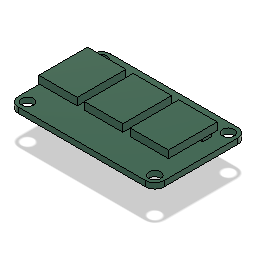
Button_PCB (Autodesk Fusion 360 design; units mm, degrees)
Autodesk Fusion 360 part; units mm, degrees
sketch "Sketch1" plane through (0, 0, 0) normal (0, 1, 0) x (1, 0, 0)
  line L0 (8.7286, -24.1072) -> (8.8714, -24.1548)
  line L1 (8.8714, -24.1548) -> (9.1095, -24.1548)
  line L2 (9.1095, -24.1548) -> (9.2048, -24.1072)
  line L3 (9.2048, -24.1072) -> (9.2524, -24.0595)
  line L4 (9.2524, -24.0595) -> (9.3, -23.9643)
  line L5 (9.3, -23.9643) -> (9.3, -23.8691)
  line L6 (9.3, -23.8691) -> (9.2524, -23.7738)
  line L7 (9.2524, -23.7738) -> (9.2048, -23.7262)
  line L8 (9.2048, -23.7262) -> (9.1095, -23.6786)
  line L9 (9.1095, -23.6786) -> (8.919, -23.631)
  line L10 (8.919, -23.631) -> (8.8238, -23.5833)
  line L11 (8.8238, -23.5833) -> (8.7762, -23.5357)
  line L12 (8.7762, -23.5357) -> (8.7286, -23.4405)
  line L13 (8.7286, -23.4405) -> (8.7286, -23.3453)
  line L14 (8.7286, -23.3453) -> (8.7762, -23.25)
  line L15 (8.7762, -23.25) -> (8.8238, -23.2024)
  line L16 (8.8238, -23.2024) -> (8.919, -23.1548)
  line L17 (8.919, -23.1548) -> (9.1571, -23.1548)
  line L18 (9.1571, -23.1548) -> (9.3, -23.2024)
  line L19 (10.1571, -23.4881) -> (10.1571, -24.1548)
  line L20 (9.7286, -23.4881) -> (9.7286, -24.0119)
  line L21 (9.7286, -24.0119) -> (9.7762, -24.1072)
  line L22 (9.7762, -24.1072) -> (9.8714, -24.1548)
  line L23 (9.8714, -24.1548) -> (10.0143, -24.1548)
  line L24 (10.0143, -24.1548) -> (10.1095, -24.1072)
  line L25 (10.1095, -24.1072) -> (10.1571, -24.0595)
  line L26 (10.6333, -23.4881) -> (10.6333, -24.1548)
  line L27 (10.6333, -23.5833) -> (10.681, -23.5357)
  line L28 (10.681, -23.5357) -> (10.7762, -23.4881)
  line L29 (10.7762, -23.4881) -> (10.919, -23.4881)
  line L30 (10.919, -23.4881) -> (11.0143, -23.5357)
  line L31 (11.0143, -23.5357) -> (11.0619, -23.631)
  line L32 (11.0619, -23.631) -> (11.0619, -24.1548)
  line L33 (11.5381, -24.1548) -> (11.5381, -23.4881)
  line L34 (11.5381, -23.6786) -> (11.5857, -23.5833)
  line L35 (11.5857, -23.5833) -> (11.6333, -23.5357)
  line L36 (11.6333, -23.5357) -> (11.7286, -23.4881)
  line L37 (11.7286, -23.4881) -> (11.8238, -23.4881)
  line L38 (12.1571, -24.1548) -> (12.1571, -23.4881)
  line L39 (12.1571, -23.1548) -> (12.1095, -23.2024)
  line L40 (12.1095, -23.2024) -> (12.1571, -23.25)
  line L41 (12.1571, -23.25) -> (12.2048, -23.2024)
  line L42 (12.2048, -23.2024) -> (12.1571, -23.1548)
  line L43 (12.1571, -23.1548) -> (12.1571, -23.25)
  line L44 (12.5857, -24.1072) -> (12.681, -24.1548)
  line L45 (12.681, -24.1548) -> (12.8714, -24.1548)
  line L46 (12.8714, -24.1548) -> (12.9667, -24.1072)
  line L47 (12.9667, -24.1072) -> (13.0143, -24.0119)
  line L48 (13.0143, -24.0119) -> (13.0143, -23.9643)
  line L49 (13.0143, -23.9643) -> (12.9667, -23.8691)
  line L50 (12.9667, -23.8691) -> (12.8714, -23.8214)
  line L51 (12.8714, -23.8214) -> (12.7286, -23.8214)
  line L52 (12.7286, -23.8214) -> (12.6333, -23.7738)
  line L53 (12.6333, -23.7738) -> (12.5857, -23.6786)
  line L54 (12.5857, -23.6786) -> (12.5857, -23.631)
  line L55 (12.5857, -23.631) -> (12.6333, -23.5357)
  line L56 (12.6333, -23.5357) -> (12.7286, -23.4881)
  line L57 (12.7286, -23.4881) -> (12.8714, -23.4881)
  line L58 (12.8714, -23.4881) -> (12.9667, -23.5357)
  line L59 (13.8238, -24.1072) -> (13.7286, -24.1548)
  line L60 (13.7286, -24.1548) -> (13.5381, -24.1548)
  line L61 (13.5381, -24.1548) -> (13.4429, -24.1072)
  line L62 (13.4429, -24.1072) -> (13.3952, -24.0119)
  line L63 (13.3952, -24.0119) -> (13.3952, -23.631)
  line L64 (13.3952, -23.631) -> (13.4429, -23.5357)
  line L65 (13.4429, -23.5357) -> (13.5381, -23.4881)
  line L66 (13.5381, -23.4881) -> (13.7286, -23.4881)
  line L67 (13.7286, -23.4881) -> (13.8238, -23.5357)
  line L68 (13.8238, -23.5357) -> (13.8714, -23.631)
  line L69 (13.8714, -23.631) -> (13.8714, -23.7262)
  line L70 (13.8714, -23.7262) -> (13.3952, -23.8214)
  line L71 (15.0143, -23.8691) -> (15.4905, -23.8691)
  line L72 (14.919, -24.1548) -> (15.2524, -23.1548)
  line L73 (15.2524, -23.1548) -> (15.5857, -24.1548)
  line L74 (16.0619, -24.1548) -> (15.9667, -24.1072)
  line L75 (15.9667, -24.1072) -> (15.919, -24.0119)
  line L76 (15.919, -24.0119) -> (15.919, -23.1548)
  line L77 (16.8714, -24.1548) -> (16.8714, -23.631)
  line L78 (16.8714, -23.631) -> (16.8238, -23.5357)
  line L79 (16.8238, -23.5357) -> (16.7286, -23.4881)
  line L80 (16.7286, -23.4881) -> (16.5381, -23.4881)
  line L81 (16.5381, -23.4881) -> (16.4429, -23.5357)
  line L82 (16.8714, -24.1072) -> (16.7762, -24.1548)
  line L83 (16.7762, -24.1548) -> (16.5381, -24.1548)
  line L84 (16.5381, -24.1548) -> (16.4429, -24.1072)
  line L85 (16.4429, -24.1072) -> (16.3952, -24.0119)
  line L86 (16.3952, -24.0119) -> (16.3952, -23.9167)
  line L87 (16.3952, -23.9167) -> (16.4429, -23.8214)
  line L88 (16.4429, -23.8214) -> (16.5381, -23.7738)
  line L89 (16.5381, -23.7738) -> (16.7762, -23.7738)
  line L90 (16.7762, -23.7738) -> (16.8714, -23.7262)
  line L91 (17.3476, -24.1548) -> (17.3476, -23.4881)
  line L92 (17.3476, -23.6786) -> (17.3952, -23.5833)
  line L93 (17.3952, -23.5833) -> (17.4429, -23.5357)
  line L94 (17.4429, -23.5357) -> (17.5381, -23.4881)
  line L95 (17.5381, -23.4881) -> (17.6333, -23.4881)
  line L96 (17.9667, -24.1548) -> (17.9667, -23.4881)
  line L97 (17.9667, -23.5833) -> (18.0143, -23.5357)
  line L98 (18.0143, -23.5357) -> (18.1095, -23.4881)
  line L99 (18.1095, -23.4881) -> (18.2524, -23.4881)
  line L100 (18.2524, -23.4881) -> (18.3476, -23.5357)
  line L101 (18.3476, -23.5357) -> (18.3952, -23.631)
  line L102 (18.3952, -23.631) -> (18.3952, -24.1548)
  line L103 (18.3952, -23.631) -> (18.4429, -23.5357)
  line L104 (18.4429, -23.5357) -> (18.5381, -23.4881)
  line L105 (18.5381, -23.4881) -> (18.681, -23.4881)
  line L106 (18.681, -23.4881) -> (18.7762, -23.5357)
  line L107 (18.7762, -23.5357) -> (18.8238, -23.631)
  line L108 (18.8238, -23.631) -> (18.8238, -24.1548)
  line L109 (19.919, -23.1548) -> (20.2524, -24.1548)
  line L110 (20.2524, -24.1548) -> (20.5857, -23.1548)
  line L111 (20.8238, -23.1548) -> (21.4429, -23.1548)
  line L112 (21.4429, -23.1548) -> (21.1095, -23.5357)
  line L113 (21.1095, -23.5357) -> (21.2524, -23.5357)
  line L114 (21.2524, -23.5357) -> (21.3476, -23.5833)
  line L115 (21.3476, -23.5833) -> (21.3952, -23.631)
  line L116 (21.3952, -23.631) -> (21.4429, -23.7262)
  line L117 (21.4429, -23.7262) -> (21.4429, -23.9643)
  line L118 (21.4429, -23.9643) -> (21.3952, -24.0595)
  line L119 (21.3952, -24.0595) -> (21.3476, -24.1072)
  line L120 (21.3476, -24.1072) -> (21.2524, -24.1548)
  line L121 (21.2524, -24.1548) -> (20.9667, -24.1548)
  line L122 (20.9667, -24.1548) -> (20.8714, -24.1072)
  line L123 (20.8714, -24.1072) -> (20.8238, -24.0595)
  line L124 (21.8714, -24.0595) -> (21.919, -24.1072)
  line L125 (21.919, -24.1072) -> (21.8714, -24.1548)
  line L126 (21.8714, -24.1548) -> (21.8238, -24.1072)
  line L127 (21.8238, -24.1072) -> (21.8714, -24.0595)
  line L128 (21.8714, -24.0595) -> (21.8714, -24.1548)
  line L129 (21.8714, -23.5357) -> (21.919, -23.5833)
  line L130 (21.919, -23.5833) -> (21.8714, -23.631)
  line L131 (21.8714, -23.631) -> (21.8238, -23.5833)
  line L132 (21.8238, -23.5833) -> (21.8714, -23.5357)
  line L133 (21.8714, -23.5357) -> (21.8714, -23.631)
  line L134 (23.4429, -23.631) -> (23.5857, -23.6786)
  line L135 (23.5857, -23.6786) -> (23.6333, -23.7262)
  line L136 (23.6333, -23.7262) -> (23.681, -23.8214)
  line L137 (23.681, -23.8214) -> (23.681, -23.9643)
  line L138 (23.681, -23.9643) -> (23.6333, -24.0595)
  line L139 (23.6333, -24.0595) -> (23.5857, -24.1072)
  line L140 (23.5857, -24.1072) -> (23.4905, -24.1548)
  line L141 (23.4905, -24.1548) -> (23.1095, -24.1548)
  line L142 (23.1095, -24.1548) -> (23.1095, -23.1548)
  line L143 (23.1095, -23.1548) -> (23.4429, -23.1548)
  line L144 (23.4429, -23.1548) -> (23.5381, -23.2024)
  line L145 (23.5381, -23.2024) -> (23.5857, -23.25)
  line L146 (23.5857, -23.25) -> (23.6333, -23.3453)
  line L147 (23.6333, -23.3453) -> (23.6333, -23.4405)
  line L148 (23.6333, -23.4405) -> (23.5857, -23.5357)
  line L149 (23.5857, -23.5357) -> (23.5381, -23.5833)
  line L150 (23.5381, -23.5833) -> (23.4429, -23.631)
  line L151 (23.4429, -23.631) -> (23.1095, -23.631)
  line L152 (24.5381, -23.4881) -> (24.5381, -24.1548)
  line L153 (24.1095, -23.4881) -> (24.1095, -24.0119)
  line L154 (24.1095, -24.0119) -> (24.1571, -24.1072)
  line L155 (24.1571, -24.1072) -> (24.2524, -24.1548)
  line L156 (24.2524, -24.1548) -> (24.3952, -24.1548)
  line L157 (24.3952, -24.1548) -> (24.4905, -24.1072)
  line L158 (24.4905, -24.1072) -> (24.5381, -24.0595)
  line L159 (24.8714, -23.4881) -> (25.2524, -23.4881)
  line L160 (25.0143, -23.1548) -> (25.0143, -24.0119)
  line L161 (25.0143, -24.0119) -> (25.0619, -24.1072)
  line L162 (25.0619, -24.1072) -> (25.1571, -24.1548)
  line L163 (25.1571, -24.1548) -> (25.2524, -24.1548)
  line L164 (25.4429, -23.4881) -> (25.8238, -23.4881)
  line L165 (25.5857, -23.1548) -> (25.5857, -24.0119)
  line L166 (25.5857, -24.0119) -> (25.6333, -24.1072)
  line L167 (25.6333, -24.1072) -> (25.7286, -24.1548)
  line L168 (25.7286, -24.1548) -> (25.8238, -24.1548)
  line L169 (26.3, -24.1548) -> (26.2048, -24.1072)
  line L170 (26.2048, -24.1072) -> (26.1571, -24.0595)
  line L171 (26.1571, -24.0595) -> (26.1095, -23.9643)
  line L172 (26.1095, -23.9643) -> (26.1095, -23.6786)
  line L173 (26.1095, -23.6786) -> (26.1571, -23.5833)
  line L174 (26.1571, -23.5833) -> (26.2048, -23.5357)
  line L175 (26.2048, -23.5357) -> (26.3, -23.4881)
  line L176 (26.3, -23.4881) -> (26.4429, -23.4881)
  line L177 (26.4429, -23.4881) -> (26.5381, -23.5357)
  line L178 (26.5381, -23.5357) -> (26.5857, -23.5833)
  line L179 (26.5857, -23.5833) -> (26.6333, -23.6786)
  line L180 (26.6333, -23.6786) -> (26.6333, -23.9643)
  line L181 (26.6333, -23.9643) -> (26.5857, -24.0595)
  line L182 (26.5857, -24.0595) -> (26.5381, -24.1072)
  line L183 (26.5381, -24.1072) -> (26.4429, -24.1548)
  line L184 (26.4429, -24.1548) -> (26.3, -24.1548)
  line L185 (27.0619, -23.4881) -> (27.0619, -24.1548)
  line L186 (27.0619, -23.5833) -> (27.1095, -23.5357)
  line L187 (27.1095, -23.5357) -> (27.2048, -23.4881)
  line L188 (27.2048, -23.4881) -> (27.3476, -23.4881)
  line L189 (27.3476, -23.4881) -> (27.4429, -23.5357)
  line L190 (27.4429, -23.5357) -> (27.4905, -23.631)
  line L191 (27.4905, -23.631) -> (27.4905, -24.1548)
  line L192 (28.7286, -24.1548) -> (28.7286, -23.1548)
  line L193 (28.7286, -23.1548) -> (29.1095, -23.1548)
  line L194 (29.1095, -23.1548) -> (29.2048, -23.2024)
  line L195 (29.2048, -23.2024) -> (29.2524, -23.25)
  line L196 (29.2524, -23.25) -> (29.3, -23.3453)
  line L197 (29.3, -23.3453) -> (29.3, -23.4881)
  line L198 (29.3, -23.4881) -> (29.2524, -23.5833)
  line L199 (29.2524, -23.5833) -> (29.2048, -23.631)
  line L200 (29.2048, -23.631) -> (29.1095, -23.6786)
  line L201 (29.1095, -23.6786) -> (28.7286, -23.6786)
  line L202 (30.3, -24.0595) -> (30.2524, -24.1072)
  line L203 (30.2524, -24.1072) -> (30.1095, -24.1548)
  line L204 (30.1095, -24.1548) -> (30.0143, -24.1548)
  line L205 (30.0143, -24.1548) -> (29.8714, -24.1072)
  line L206 (29.8714, -24.1072) -> (29.7762, -24.0119)
  line L207 (29.7762, -24.0119) -> (29.7286, -23.9167)
  line L208 (29.7286, -23.9167) -> (29.681, -23.7262)
  line L209 (29.681, -23.7262) -> (29.681, -23.5833)
  line L210 (29.681, -23.5833) -> (29.7286, -23.3929)
  line L211 (29.7286, -23.3929) -> (29.7762, -23.2976)
  line L212 (29.7762, -23.2976) -> (29.8714, -23.2024)
  line L213 (29.8714, -23.2024) -> (30.0143, -23.1548)
  line L214 (30.0143, -23.1548) -> (30.1095, -23.1548)
  line L215 (30.1095, -23.1548) -> (30.2524, -23.2024)
  line L216 (30.2524, -23.2024) -> (30.3, -23.25)
  line L217 (31.0619, -23.631) -> (31.2048, -23.6786)
  line L218 (31.2048, -23.6786) -> (31.2524, -23.7262)
  line L219 (31.2524, -23.7262) -> (31.3, -23.8214)
  line L220 (31.3, -23.8214) -> (31.3, -23.9643)
  line L221 (31.3, -23.9643) -> (31.2524, -24.0595)
  line L222 (31.2524, -24.0595) -> (31.2048, -24.1072)
  line L223 (31.2048, -24.1072) -> (31.1095, -24.1548)
  line L224 (31.1095, -24.1548) -> (30.7286, -24.1548)
  line L225 (30.7286, -24.1548) -> (30.7286, -23.1548)
  line L226 (30.7286, -23.1548) -> (31.0619, -23.1548)
  line L227 (31.0619, -23.1548) -> (31.1571, -23.2024)
  line L228 (31.1571, -23.2024) -> (31.2048, -23.25)
  line L229 (31.2048, -23.25) -> (31.2524, -23.3453)
  line L230 (31.2524, -23.3453) -> (31.2524, -23.4405)
  line L231 (31.2524, -23.4405) -> (31.2048, -23.5357)
  line L232 (31.2048, -23.5357) -> (31.1571, -23.5833)
  line L233 (31.1571, -23.5833) -> (31.0619, -23.631)
  line L234 (31.0619, -23.631) -> (30.7286, -23.631)
  line L235 (32.3476, -23.1548) -> (32.681, -24.1548)
  line L236 (32.681, -24.1548) -> (33.0143, -23.1548)
  line L237 (33.8714, -24.1548) -> (33.3, -24.1548)
  line L238 (33.5857, -24.1548) -> (33.5857, -23.1548)
  line L239 (33.5857, -23.1548) -> (33.4905, -23.2976)
  line L240 (33.4905, -23.2976) -> (33.3952, -23.3929)
  line L241 (33.3952, -23.3929) -> (33.3, -23.4405)
  line L242 (7.7167, -13.6348) -> (7.7167, -14.3491)
  line L243 (7.7167, -14.3491) -> (7.669, -14.4919)
  line L244 (7.669, -14.4919) -> (7.5738, -14.5872)
  line L245 (7.5738, -14.5872) -> (7.431, -14.6348)
  line L246 (7.431, -14.6348) -> (7.3357, -14.6348)
  line L247 (8.6214, -13.9681) -> (8.6214, -14.6348)
  line L248 (8.3833, -13.5872) -> (8.1452, -14.3014)
  line L249 (8.1452, -14.3014) -> (8.7643, -14.3014)
  line L250 (3.8833, -16.1348) -> (3.4071, -16.1348)
  line L251 (3.4071, -16.1348) -> (3.4071, -15.1348)
  line L252 (4.2167, -15.611) -> (4.55, -15.611)
  line L253 (4.6929, -16.1348) -> (4.2167, -16.1348)
  line L254 (4.2167, -16.1348) -> (4.2167, -15.1348)
  line L255 (4.2167, -15.1348) -> (4.6929, -15.1348)
  line L256 (5.4548, -15.611) -> (5.1214, -15.611)
  line L257 (5.1214, -16.1348) -> (5.1214, -15.1348)
  line L258 (5.1214, -15.1348) -> (5.5976, -15.1348)
  line L259 (5.8357, -15.1348) -> (6.4071, -15.1348)
  line L260 (6.1214, -16.1348) -> (6.1214, -15.1348)
  line L261 (6.5024, -16.23) -> (7.2643, -16.23)
  line L262 (7.8357, -15.611) -> (7.9786, -15.6586)
  line L263 (7.9786, -15.6586) -> (8.0262, -15.7062)
  line L264 (8.0262, -15.7062) -> (8.0738, -15.8014)
  line L265 (8.0738, -15.8014) -> (8.0738, -15.9443)
  line L266 (8.0738, -15.9443) -> (8.0262, -16.0395)
  line L267 (8.0262, -16.0395) -> (7.9786, -16.0872)
  line L268 (7.9786, -16.0872) -> (7.8833, -16.1348)
  line L269 (7.8833, -16.1348) -> (7.5024, -16.1348)
  line L270 (7.5024, -16.1348) -> (7.5024, -15.1348)
  line L271 (7.5024, -15.1348) -> (7.8357, -15.1348)
  line L272 (7.8357, -15.1348) -> (7.931, -15.1824)
  line L273 (7.931, -15.1824) -> (7.9786, -15.23)
  line L274 (7.9786, -15.23) -> (8.0262, -15.3253)
  line L275 (8.0262, -15.3253) -> (8.0262, -15.4205)
  line L276 (8.0262, -15.4205) -> (7.9786, -15.5157)
  line L277 (7.9786, -15.5157) -> (7.931, -15.5633)
  line L278 (7.931, -15.5633) -> (7.8357, -15.611)
  line L279 (7.8357, -15.611) -> (7.5024, -15.611)
  line L280 (8.5024, -15.1348) -> (8.5024, -15.9443)
  line L281 (8.5024, -15.9443) -> (8.55, -16.0395)
  line L282 (8.55, -16.0395) -> (8.5976, -16.0872)
  line L283 (8.5976, -16.0872) -> (8.6929, -16.1348)
  line L284 (8.6929, -16.1348) -> (8.8833, -16.1348)
  line L285 (8.8833, -16.1348) -> (8.9786, -16.0872)
  line L286 (8.9786, -16.0872) -> (9.0262, -16.0395)
  line L287 (9.0262, -16.0395) -> (9.0738, -15.9443)
  line L288 (9.0738, -15.9443) -> (9.0738, -15.1348)
  line L289 (9.4071, -15.1348) -> (9.9786, -15.1348)
  line L290 (9.6929, -16.1348) -> (9.6929, -15.1348)
  line L291 (10.169, -15.1348) -> (10.7405, -15.1348)
  line L292 (10.4548, -16.1348) -> (10.4548, -15.1348)
  line L293 (11.2643, -15.1348) -> (11.4548, -15.1348)
  line L294 (11.4548, -15.1348) -> (11.55, -15.1824)
  line L295 (11.55, -15.1824) -> (11.6452, -15.2776)
  line L296 (11.6452, -15.2776) -> (11.6929, -15.4681)
  line L297 (11.6929, -15.4681) -> (11.6929, -15.8014)
  line L298 (11.6929, -15.8014) -> (11.6452, -15.9919)
  line L299 (11.6452, -15.9919) -> (11.55, -16.0872)
  line L300 (11.55, -16.0872) -> (11.4548, -16.1348)
  line L301 (11.4548, -16.1348) -> (11.2643, -16.1348)
  line L302 (11.2643, -16.1348) -> (11.169, -16.0872)
  line L303 (11.169, -16.0872) -> (11.0738, -15.9919)
  line L304 (11.0738, -15.9919) -> (11.0262, -15.8014)
  line L305 (11.0262, -15.8014) -> (11.0262, -15.4681)
  line L306 (11.0262, -15.4681) -> (11.0738, -15.2776)
  line L307 (11.0738, -15.2776) -> (11.169, -15.1824)
  line L308 (11.169, -15.1824) -> (11.2643, -15.1348)
  line L309 (12.1214, -16.1348) -> (12.1214, -15.1348)
  line L310 (12.1214, -15.1348) -> (12.6929, -16.1348)
  line L311 (12.6929, -16.1348) -> (12.6929, -15.1348)
  line L312 (34.3167, -13.6348) -> (34.3167, -14.3491)
  line L313 (34.3167, -14.3491) -> (34.269, -14.4919)
  line L314 (34.269, -14.4919) -> (34.1738, -14.5872)
  line L315 (34.1738, -14.5872) -> (34.031, -14.6348)
  line L316 (34.031, -14.6348) -> (33.9357, -14.6348)
  line L317 (34.7452, -13.73) -> (34.7929, -13.6824)
  line L318 (34.7929, -13.6824) -> (34.8881, -13.6348)
  line L319 (34.8881, -13.6348) -> (35.1262, -13.6348)
  line L320 (35.1262, -13.6348) -> (35.2214, -13.6824)
  line L321 (35.2214, -13.6824) -> (35.269, -13.73)
  line L322 (35.269, -13.73) -> (35.3167, -13.8253)
  line L323 (35.3167, -13.8253) -> (35.3167, -13.9205)
  line L324 (35.3167, -13.9205) -> (35.269, -14.0633)
  line L325 (35.269, -14.0633) -> (34.6976, -14.6348)
  line L326 (34.6976, -14.6348) -> (35.3167, -14.6348)
  line L327 (30.1024, -16.1348) -> (29.769, -15.6586)
  line L328 (29.531, -16.1348) -> (29.531, -15.1348)
  line L329 (29.531, -15.1348) -> (29.9119, -15.1348)
  line L330 (29.9119, -15.1348) -> (30.0071, -15.1824)
  line L331 (30.0071, -15.1824) -> (30.0548, -15.23)
  line L332 (30.0548, -15.23) -> (30.1024, -15.3253)
  line L333 (30.1024, -15.3253) -> (30.1024, -15.4681)
  line L334 (30.1024, -15.4681) -> (30.0548, -15.5633)
  line L335 (30.0548, -15.5633) -> (30.0071, -15.611)
  line L336 (30.0071, -15.611) -> (29.9119, -15.6586)
  line L337 (29.9119, -15.6586) -> (29.531, -15.6586)
  line L338 (30.531, -16.1348) -> (30.531, -15.1348)
  line L339 (31.531, -15.1824) -> (31.4357, -15.1348)
  line L340 (31.4357, -15.1348) -> (31.2929, -15.1348)
  line L341 (31.2929, -15.1348) -> (31.15, -15.1824)
  line L342 (31.15, -15.1824) -> (31.0548, -15.2776)
  line L343 (31.0548, -15.2776) -> (31.0071, -15.3729)
  line L344 (31.0071, -15.3729) -> (30.9595, -15.5633)
  line L345 (30.9595, -15.5633) -> (30.9595, -15.7062)
  line L346 (30.9595, -15.7062) -> (31.0071, -15.8967)
  line L347 (31.0071, -15.8967) -> (31.0548, -15.9919)
  line L348 (31.0548, -15.9919) -> (31.15, -16.0872)
  line L349 (31.15, -16.0872) -> (31.2929, -16.1348)
  line L350 (31.2929, -16.1348) -> (31.3881, -16.1348)
  line L351 (31.3881, -16.1348) -> (31.531, -16.0872)
  line L352 (31.531, -16.0872) -> (31.5786, -16.0395)
  line L353 (31.5786, -16.0395) -> (31.5786, -15.7062)
  line L354 (31.5786, -15.7062) -> (31.3881, -15.7062)
  line L355 (32.0071, -16.1348) -> (32.0071, -15.1348)
  line L356 (32.0071, -15.611) -> (32.5786, -15.611)
  line L357 (32.5786, -16.1348) -> (32.5786, -15.1348)
  line L358 (32.9119, -15.1348) -> (33.4833, -15.1348)
  line L359 (33.1976, -16.1348) -> (33.1976, -15.1348)
  line L360 (33.5786, -16.23) -> (34.3405, -16.23)
  line L361 (34.9119, -15.611) -> (35.0548, -15.6586)
  line L362 (35.0548, -15.6586) -> (35.1024, -15.7062)
  line L363 (35.1024, -15.7062) -> (35.15, -15.8014)
  line L364 (35.15, -15.8014) -> (35.15, -15.9443)
  line L365 (35.15, -15.9443) -> (35.1024, -16.0395)
  line L366 (35.1024, -16.0395) -> (35.0548, -16.0872)
  line L367 (35.0548, -16.0872) -> (34.9595, -16.1348)
  line L368 (34.9595, -16.1348) -> (34.5786, -16.1348)
  line L369 (34.5786, -16.1348) -> (34.5786, -15.1348)
  line L370 (34.5786, -15.1348) -> (34.9119, -15.1348)
  line L371 (34.9119, -15.1348) -> (35.0071, -15.1824)
  line L372 (35.0071, -15.1824) -> (35.0548, -15.23)
  line L373 (35.0548, -15.23) -> (35.1024, -15.3253)
  line L374 (35.1024, -15.3253) -> (35.1024, -15.4205)
  line L375 (35.1024, -15.4205) -> (35.0548, -15.5157)
  line L376 (35.0548, -15.5157) -> (35.0071, -15.5633)
  line L377 (35.0071, -15.5633) -> (34.9119, -15.611)
  line L378 (34.9119, -15.611) -> (34.5786, -15.611)
  line L379 (35.5786, -15.1348) -> (35.5786, -15.9443)
  line L380 (35.5786, -15.9443) -> (35.6262, -16.0395)
  line L381 (35.6262, -16.0395) -> (35.6738, -16.0872)
  line L382 (35.6738, -16.0872) -> (35.769, -16.1348)
  line L383 (35.769, -16.1348) -> (35.9595, -16.1348)
  line L384 (35.9595, -16.1348) -> (36.0548, -16.0872)
  line L385 (36.0548, -16.0872) -> (36.1024, -16.0395)
  line L386 (36.1024, -16.0395) -> (36.15, -15.9443)
  line L387 (36.15, -15.9443) -> (36.15, -15.1348)
  line L388 (36.4833, -15.1348) -> (37.0548, -15.1348)
  line L389 (36.769, -16.1348) -> (36.769, -15.1348)
  line L390 (37.2452, -15.1348) -> (37.8167, -15.1348)
  line L391 (37.531, -16.1348) -> (37.531, -15.1348)
  line L392 (38.3405, -15.1348) -> (38.531, -15.1348)
  line L393 (38.531, -15.1348) -> (38.6262, -15.1824)
  line L394 (38.6262, -15.1824) -> (38.7214, -15.2776)
  line L395 (38.7214, -15.2776) -> (38.769, -15.4681)
  line L396 (38.769, -15.4681) -> (38.769, -15.8014)
  line L397 (38.769, -15.8014) -> (38.7214, -15.9919)
  line L398 (38.7214, -15.9919) -> (38.6262, -16.0872)
  line L399 (38.6262, -16.0872) -> (38.531, -16.1348)
  line L400 (38.531, -16.1348) -> (38.3405, -16.1348)
  line L401 (38.3405, -16.1348) -> (38.2452, -16.0872)
  line L402 (38.2452, -16.0872) -> (38.15, -15.9919)
  line L403 (38.15, -15.9919) -> (38.1024, -15.8014)
  line L404 (38.1024, -15.8014) -> (38.1024, -15.4681)
  line L405 (38.1024, -15.4681) -> (38.15, -15.2776)
  line L406 (38.15, -15.2776) -> (38.2452, -15.1824)
  line L407 (38.2452, -15.1824) -> (38.3405, -15.1348)
  line L408 (39.1976, -16.1348) -> (39.1976, -15.1348)
  line L409 (39.1976, -15.1348) -> (39.769, -16.1348)
  line L410 (39.769, -16.1348) -> (39.769, -15.1348)
  line L411 (21.0167, -13.6348) -> (21.0167, -14.3491)
  line L412 (21.0167, -14.3491) -> (20.969, -14.4919)
  line L413 (20.969, -14.4919) -> (20.8738, -14.5872)
  line L414 (20.8738, -14.5872) -> (20.731, -14.6348)
  line L415 (20.731, -14.6348) -> (20.6357, -14.6348)
  line L416 (21.3976, -13.6348) -> (22.0167, -13.6348)
  line L417 (22.0167, -13.6348) -> (21.6833, -14.0157)
  line L418 (21.6833, -14.0157) -> (21.8262, -14.0157)
  line L419 (21.8262, -14.0157) -> (21.9214, -14.0633)
  line L420 (21.9214, -14.0633) -> (21.969, -14.111)
  line L421 (21.969, -14.111) -> (22.0167, -14.2062)
  line L422 (22.0167, -14.2062) -> (22.0167, -14.4443)
  line L423 (22.0167, -14.4443) -> (21.969, -14.5395)
  line L424 (21.969, -14.5395) -> (21.9214, -14.5872)
  line L425 (21.9214, -14.5872) -> (21.8262, -14.6348)
  line L426 (21.8262, -14.6348) -> (21.5405, -14.6348)
  line L427 (21.5405, -14.6348) -> (21.4452, -14.5872)
  line L428 (21.4452, -14.5872) -> (21.3976, -14.5395)
  line L429 (16.2714, -16.1348) -> (16.2714, -15.1348)
  line L430 (16.2714, -15.1348) -> (16.5714, -15.8491)
  line L431 (16.5714, -15.8491) -> (16.8714, -15.1348)
  line L432 (16.8714, -15.1348) -> (16.8714, -16.1348)
  line L433 (17.3, -16.1348) -> (17.3, -15.1348)
  line L434 (17.7286, -16.1348) -> (17.7286, -15.1348)
  line L435 (17.7286, -15.1348) -> (17.9429, -15.1348)
  line L436 (17.9429, -15.1348) -> (18.0714, -15.1824)
  line L437 (18.0714, -15.1824) -> (18.1571, -15.2776)
  line L438 (18.1571, -15.2776) -> (18.2, -15.3729)
  line L439 (18.2, -15.3729) -> (18.2429, -15.5633)
  line L440 (18.2429, -15.5633) -> (18.2429, -15.7062)
  line L441 (18.2429, -15.7062) -> (18.2, -15.8967)
  line L442 (18.2, -15.8967) -> (18.1571, -15.9919)
  line L443 (18.1571, -15.9919) -> (18.0714, -16.0872)
  line L444 (18.0714, -16.0872) -> (17.9429, -16.1348)
  line L445 (17.9429, -16.1348) -> (17.7286, -16.1348)
  line L446 (18.6286, -16.1348) -> (18.6286, -15.1348)
  line L447 (18.6286, -15.1348) -> (18.8429, -15.1348)
  line L448 (18.8429, -15.1348) -> (18.9714, -15.1824)
  line L449 (18.9714, -15.1824) -> (19.0571, -15.2776)
  line L450 (19.0571, -15.2776) -> (19.1, -15.3729)
  line L451 (19.1, -15.3729) -> (19.1429, -15.5633)
  line L452 (19.1429, -15.5633) -> (19.1429, -15.7062)
  line L453 (19.1429, -15.7062) -> (19.1, -15.8967)
  line L454 (19.1, -15.8967) -> (19.0571, -15.9919)
  line L455 (19.0571, -15.9919) -> (18.9714, -16.0872)
  line L456 (18.9714, -16.0872) -> (18.8429, -16.1348)
  line L457 (18.8429, -16.1348) -> (18.6286, -16.1348)
  line L458 (19.9571, -16.1348) -> (19.5286, -16.1348)
  line L459 (19.5286, -16.1348) -> (19.5286, -15.1348)
  line L460 (20.2571, -15.611) -> (20.5571, -15.611)
  line L461 (20.6857, -16.1348) -> (20.2571, -16.1348)
  line L462 (20.2571, -16.1348) -> (20.2571, -15.1348)
  line L463 (20.2571, -15.1348) -> (20.6857, -15.1348)
  line L464 (20.8571, -16.23) -> (21.5429, -16.23)
  line L465 (22.0571, -15.611) -> (22.1857, -15.6586)
  line L466 (22.1857, -15.6586) -> (22.2286, -15.7062)
  line L467 (22.2286, -15.7062) -> (22.2714, -15.8014)
  line L468 (22.2714, -15.8014) -> (22.2714, -15.9443)
  line L469 (22.2714, -15.9443) -> (22.2286, -16.0395)
  line L470 (22.2286, -16.0395) -> (22.1857, -16.0872)
  line L471 (22.1857, -16.0872) -> (22.1, -16.1348)
  line L472 (22.1, -16.1348) -> (21.7571, -16.1348)
  line L473 (21.7571, -16.1348) -> (21.7571, -15.1348)
  line L474 (21.7571, -15.1348) -> (22.0571, -15.1348)
  line L475 (22.0571, -15.1348) -> (22.1429, -15.1824)
  line L476 (22.1429, -15.1824) -> (22.1857, -15.23)
  line L477 (22.1857, -15.23) -> (22.2286, -15.3253)
  line L478 (22.2286, -15.3253) -> (22.2286, -15.4205)
  line L479 (22.2286, -15.4205) -> (22.1857, -15.5157)
  line L480 (22.1857, -15.5157) -> (22.1429, -15.5633)
  line L481 (22.1429, -15.5633) -> (22.0571, -15.611)
  line L482 (22.0571, -15.611) -> (21.7571, -15.611)
  line L483 (22.6571, -15.1348) -> (22.6571, -15.9443)
  line L484 (22.6571, -15.9443) -> (22.7, -16.0395)
  line L485 (22.7, -16.0395) -> (22.7429, -16.0872)
  line L486 (22.7429, -16.0872) -> (22.8286, -16.1348)
  line L487 (22.8286, -16.1348) -> (23, -16.1348)
  line L488 (23, -16.1348) -> (23.0857, -16.0872)
  line L489 (23.0857, -16.0872) -> (23.1286, -16.0395)
  line L490 (23.1286, -16.0395) -> (23.1714, -15.9443)
  line L491 (23.1714, -15.9443) -> (23.1714, -15.1348)
  line L492 (23.4714, -15.1348) -> (23.9857, -15.1348)
  line L493 (23.7286, -16.1348) -> (23.7286, -15.1348)
  line L494 (24.1571, -15.1348) -> (24.6714, -15.1348)
  line L495 (24.4143, -16.1348) -> (24.4143, -15.1348)
  line L496 (25.1429, -15.1348) -> (25.3143, -15.1348)
  line L497 (25.3143, -15.1348) -> (25.4, -15.1824)
  line L498 (25.4, -15.1824) -> (25.4857, -15.2776)
  line L499 (25.4857, -15.2776) -> (25.5286, -15.4681)
  line L500 (25.5286, -15.4681) -> (25.5286, -15.8014)
  line L501 (25.5286, -15.8014) -> (25.4857, -15.9919)
  line L502 (25.4857, -15.9919) -> (25.4, -16.0872)
  line L503 (25.4, -16.0872) -> (25.3143, -16.1348)
  line L504 (25.3143, -16.1348) -> (25.1429, -16.1348)
  line L505 (25.1429, -16.1348) -> (25.0571, -16.0872)
  line L506 (25.0571, -16.0872) -> (24.9714, -15.9919)
  line L507 (24.9714, -15.9919) -> (24.9286, -15.8014)
  line L508 (24.9286, -15.8014) -> (24.9286, -15.4681)
  line L509 (24.9286, -15.4681) -> (24.9714, -15.2776)
  line L510 (24.9714, -15.2776) -> (25.0571, -15.1824)
  line L511 (25.0571, -15.1824) -> (25.1429, -15.1348)
  line L512 (25.9143, -16.1348) -> (25.9143, -15.1348)
  line L513 (25.9143, -15.1348) -> (26.4286, -16.1348)
  line L514 (26.4286, -16.1348) -> (26.4286, -15.1348)
  line L515 (8, -6.37) -> (13.6, -6.37)
  line L516 (8, -7.6) -> (8, -6.37)
  line L517 (13.6, -6.37) -> (2.4, -6.37)
  line L518 (2.4, -6.37) -> (2.4, -20.57)
  line L519 (2.4, -20.57) -> (13.6, -20.57)
  line L520 (13.6, -20.57) -> (13.6, -6.37)
  line L521 (34.6, -6.37) -> (40.2, -6.37)
  line L522 (34.6, -7.6) -> (34.6, -6.37)
  line L523 (40.2, -6.37) -> (29, -6.37)
  line L524 (29, -6.37) -> (29, -20.57)
  line L525 (29, -20.57) -> (40.2, -20.57)
  line L526 (40.2, -20.57) -> (40.2, -6.37)
  line L527 (21.3, -6.37) -> (26.9, -6.37)
  line L528 (21.3, -7.6) -> (21.3, -6.37)
  line L529 (26.9, -6.37) -> (15.7, -6.37)
  line L530 (15.7, -6.37) -> (15.7, -20.57)
  line L531 (15.7, -20.57) -> (26.9, -20.57)
  line L532 (26.9, -20.57) -> (26.9, -6.37)
  line L533 (21.3, -0.05) -> (39.85, -0.05)
  line L534 (0.05, -24.2) -> (0.05, -2.75)
  arc A0 (2.75, -26.9) -> (0.05, -24.2) centre (2.75, -24.2) cw
  line L535 (42.55, -2.75) -> (42.55, -24.2)
  line L536 (2.75, -0.05) -> (21.3, -0.05)
  arc A1 (0.05, -2.75) -> (2.75, -0.05) centre (2.75, -2.75) cw
  arc A2 (42.55, -24.2) -> (39.85, -26.9) centre (39.85, -24.2) cw
  circle A3 centre (2.75, -2.75) radius 1.7
  circle A4 centre (2.75, -24.2) radius 1.7
  line L537 (39.85, -26.9) -> (2.75, -26.9)
  arc A5 (39.85, -0.05) -> (42.55, -2.75) centre (39.85, -2.75) cw
  circle A6 centre (39.85, -2.75) radius 1.7
  circle A7 centre (39.85, -24.2) radius 1.7
  line L538 (21.6429, -4.7048) -> (21.9095, -4.2286)
  line L539 (22.1, -4.7048) -> (22.1, -3.7048)
  line L540 (22.1, -3.7048) -> (21.7952, -3.7048)
  line L541 (21.7952, -3.7048) -> (21.719, -3.7524)
  line L542 (21.719, -3.7524) -> (21.681, -3.8)
  line L543 (21.681, -3.8) -> (21.6429, -3.8953)
  line L544 (21.6429, -3.8953) -> (21.6429, -4.0381)
  line L545 (21.6429, -4.0381) -> (21.681, -4.1333)
  line L546 (21.681, -4.1333) -> (21.719, -4.181)
  line L547 (21.719, -4.181) -> (21.7952, -4.2286)
  line L548 (21.7952, -4.2286) -> (22.1, -4.2286)
  line L549 (21.3, -4.7048) -> (21.3, -3.7048)
  line L550 (20.5, -3.7524) -> (20.5762, -3.7048)
  line L551 (20.5762, -3.7048) -> (20.6905, -3.7048)
  line L552 (20.6905, -3.7048) -> (20.8048, -3.7524)
  line L553 (20.8048, -3.7524) -> (20.881, -3.8476)
  line L554 (20.881, -3.8476) -> (20.919, -3.9429)
  line L555 (20.919, -3.9429) -> (20.9571, -4.1333)
  line L556 (20.9571, -4.1333) -> (20.9571, -4.2762)
  line L557 (20.9571, -4.2762) -> (20.919, -4.4667)
  line L558 (20.919, -4.4667) -> (20.881, -4.5619)
  line L559 (20.881, -4.5619) -> (20.8048, -4.6572)
  line L560 (20.8048, -4.6572) -> (20.6905, -4.7048)
  line L561 (20.6905, -4.7048) -> (20.6143, -4.7048)
  line L562 (20.6143, -4.7048) -> (20.5, -4.6572)
  line L563 (20.5, -4.6572) -> (20.4619, -4.6095)
  line L564 (20.4619, -4.6095) -> (20.4619, -4.2762)
  line L565 (20.4619, -4.2762) -> (20.6143, -4.2762)
  line L566 (24.4395, -3.7624) -> (24.5157, -3.7148)
  line L567 (24.5157, -3.7148) -> (24.63, -3.7148)
  line L568 (24.63, -3.7148) -> (24.7443, -3.7624)
  line L569 (24.7443, -3.7624) -> (24.8205, -3.8576)
  line L570 (24.8205, -3.8576) -> (24.8586, -3.9529)
  line L571 (24.8586, -3.9529) -> (24.8967, -4.1433)
  line L572 (24.8967, -4.1433) -> (24.8967, -4.2862)
  line L573 (24.8967, -4.2862) -> (24.8586, -4.4767)
  line L574 (24.8586, -4.4767) -> (24.8205, -4.5719)
  line L575 (24.8205, -4.5719) -> (24.7443, -4.6672)
  line L576 (24.7443, -4.6672) -> (24.63, -4.7148)
  line L577 (24.63, -4.7148) -> (24.5538, -4.7148)
  line L578 (24.5538, -4.7148) -> (24.4395, -4.6672)
  line L579 (24.4395, -4.6672) -> (24.4014, -4.6195)
  line L580 (24.4014, -4.6195) -> (24.4014, -4.2862)
  line L581 (24.4014, -4.2862) -> (24.5538, -4.2862)
  line L582 (24.0586, -4.7148) -> (24.0586, -3.7148)
  line L583 (24.0586, -3.7148) -> (23.6014, -4.7148)
  line L584 (23.6014, -4.7148) -> (23.6014, -3.7148)
  line L585 (23.2205, -4.7148) -> (23.2205, -3.7148)
  line L586 (23.2205, -3.7148) -> (23.03, -3.7148)
  line L587 (23.03, -3.7148) -> (22.9157, -3.7624)
  line L588 (22.9157, -3.7624) -> (22.8395, -3.8576)
  line L589 (22.8395, -3.8576) -> (22.8014, -3.9529)
  line L590 (22.8014, -3.9529) -> (22.7633, -4.1433)
  line L591 (22.7633, -4.1433) -> (22.7633, -4.2862)
  line L592 (22.7633, -4.2862) -> (22.8014, -4.4767)
  line L593 (22.8014, -4.4767) -> (22.8395, -4.5719)
  line L594 (22.8395, -4.5719) -> (22.9157, -4.6672)
  line L595 (22.9157, -4.6672) -> (23.03, -4.7148)
  line L596 (23.03, -4.7148) -> (23.2205, -4.7148)
  line L597 (16.6771, -4.7048) -> (17.0581, -4.7048)
  line L598 (17.0581, -4.7048) -> (17.0581, -3.7048)
  line L599 (16.4105, -4.181) -> (16.1438, -4.181)
  line L600 (16.0295, -4.7048) -> (16.4105, -4.7048)
  line L601 (16.4105, -4.7048) -> (16.4105, -3.7048)
  line L602 (16.4105, -3.7048) -> (16.0295, -3.7048)
  line L603 (15.42, -4.181) -> (15.6867, -4.181)
  line L604 (15.6867, -4.7048) -> (15.6867, -3.7048)
  line L605 (15.6867, -3.7048) -> (15.3057, -3.7048)
  line L606 (27.4167, -3.7048) -> (27.15, -4.7048)
  line L607 (27.15, -4.7048) -> (26.8833, -3.7048)
  line L608 (26.1595, -4.6095) -> (26.1976, -4.6572)
  line L609 (26.1976, -4.6572) -> (26.3119, -4.7048)
  line L610 (26.3119, -4.7048) -> (26.3881, -4.7048)
  line L611 (26.3881, -4.7048) -> (26.5024, -4.6572)
  line L612 (26.5024, -4.6572) -> (26.5786, -4.5619)
  line L613 (26.5786, -4.5619) -> (26.6167, -4.4667)
  line L614 (26.6167, -4.4667) -> (26.6548, -4.2762)
  line L615 (26.6548, -4.2762) -> (26.6548, -4.1333)
  line L616 (26.6548, -4.1333) -> (26.6167, -3.9429)
  line L617 (26.6167, -3.9429) -> (26.5786, -3.8476)
  line L618 (26.5786, -3.8476) -> (26.5024, -3.7524)
  line L619 (26.5024, -3.7524) -> (26.3881, -3.7048)
  line L620 (26.3881, -3.7048) -> (26.3119, -3.7048)
  line L621 (26.3119, -3.7048) -> (26.1976, -3.7524)
  line L622 (26.1976, -3.7524) -> (26.1595, -3.8)
  line L623 (25.3595, -4.6095) -> (25.3976, -4.6572)
  line L624 (25.3976, -4.6572) -> (25.5119, -4.7048)
  line L625 (25.5119, -4.7048) -> (25.5881, -4.7048)
  line L626 (25.5881, -4.7048) -> (25.7024, -4.6572)
  line L627 (25.7024, -4.6572) -> (25.7786, -4.5619)
  line L628 (25.7786, -4.5619) -> (25.8167, -4.4667)
  line L629 (25.8167, -4.4667) -> (25.8548, -4.2762)
  line L630 (25.8548, -4.2762) -> (25.8548, -4.1333)
  line L631 (25.8548, -4.1333) -> (25.8167, -3.9429)
  line L632 (25.8167, -3.9429) -> (25.7786, -3.8476)
  line L633 (25.7786, -3.8476) -> (25.7024, -3.7524)
  line L634 (25.7024, -3.7524) -> (25.5881, -3.7048)
  line L635 (25.5881, -3.7048) -> (25.5119, -3.7048)
  line L636 (25.5119, -3.7048) -> (25.3976, -3.7524)
  line L637 (25.3976, -3.7524) -> (25.3595, -3.8)
  line L638 (19.6471, -4.7048) -> (19.6471, -3.7048)
  line L639 (19.6471, -3.7048) -> (19.3805, -4.4191)
  line L640 (19.3805, -4.4191) -> (19.1138, -3.7048)
  line L641 (19.1138, -3.7048) -> (19.1138, -4.7048)
  line L642 (18.7329, -4.7048) -> (18.7329, -3.7048)
  line L643 (18.3519, -4.7048) -> (18.3519, -3.7048)
  line L644 (18.3519, -3.7048) -> (18.1614, -3.7048)
  line L645 (18.1614, -3.7048) -> (18.0471, -3.7524)
  line L646 (18.0471, -3.7524) -> (17.971, -3.8476)
  line L647 (17.971, -3.8476) -> (17.9329, -3.9429)
  line L648 (17.9329, -3.9429) -> (17.8948, -4.1333)
  line L649 (17.8948, -4.1333) -> (17.8948, -4.2762)
  line L650 (17.8948, -4.2762) -> (17.9329, -4.4667)
  line L651 (17.9329, -4.4667) -> (17.971, -4.5619)
  line L652 (17.971, -4.5619) -> (18.0471, -4.6572)
  line L653 (18.0471, -4.6572) -> (18.1614, -4.7048)
  line L654 (18.1614, -4.7048) -> (18.3519, -4.7048)
  line L655 (29.0933, -1.6448) -> (29.0933, -2.3591)
  line L656 (29.0933, -2.3591) -> (29.141, -2.5019)
  line L657 (29.141, -2.5019) -> (29.2362, -2.5972)
  line L658 (29.2362, -2.5972) -> (29.379, -2.6448)
  line L659 (29.379, -2.6448) -> (29.4743, -2.6448)
  line L660 (28.0933, -2.6448) -> (28.6648, -2.6448)
  line L661 (28.379, -2.6448) -> (28.379, -1.6448)
  line L662 (28.379, -1.6448) -> (28.4743, -1.7876)
  line L663 (28.4743, -1.7876) -> (28.5695, -1.8829)
  line L664 (28.5695, -1.8829) -> (28.6648, -1.9305)
  line L665 (14.885, -3.53) -> (14.885, -0.87)
  line L666 (25.105, -3.53) -> (14.885, -3.53)
  line L667 (25.105, -3.53) -> (25.105, -0.87)
  line L668 (26.375, -3.53) -> (27.705, -3.53)
  line L669 (27.705, -3.53) -> (27.705, -2.2)
  line L670 (25.105, -0.87) -> (14.885, -0.87)
  line L671 (14.885, -0.87) -> (27.705, -0.87)
  line L672 (27.705, -0.87) -> (27.705, -3.53)
  line L673 (27.705, -3.53) -> (14.885, -3.53)
  line L674 (14.885, -3.53) -> (14.885, -0.87)
  line L675 (11.81, -6.37) -> (4.19, -6.37)
  line L676 (4.19, -6.37) -> (4.19, -8.83)
  line L677 (4.19, -8.83) -> (11.81, -8.83)
  line L678 (11.81, -8.83) -> (11.81, -6.37)
  line L679 (11.81, -6.37) -> (4.19, -8.83) construction
  line L680 (4.19, -6.37) -> (11.81, -8.83) construction
  line L681 (25.11, -6.37) -> (17.49, -6.37)
  line L682 (17.49, -6.37) -> (17.49, -8.83)
  line L683 (17.49, -8.83) -> (25.11, -8.83)
  line L684 (25.11, -8.83) -> (25.11, -6.37)
  line L685 (25.11, -6.37) -> (17.49, -8.83) construction
  line L686 (17.49, -6.37) -> (25.11, -8.83) construction
  line L687 (38.41, -6.37) -> (30.79, -6.37)
  line L688 (30.79, -6.37) -> (30.79, -8.83)
  line L689 (30.79, -8.83) -> (38.41, -8.83)
  line L690 (38.41, -8.83) -> (38.41, -6.37)
  line L691 (38.41, -6.37) -> (30.79, -8.83) construction
  line L692 (30.79, -6.37) -> (38.41, -8.83) construction
  point P0 (4.45, -2.75)
  point P1 (4.45, -24.2)
  point P2 (41.55, -2.75)
  point P3 (41.55, -24.2)
  point P4 (8, -7.6)
  point P5 (21.3, -7.6)
  point P6 (34.6, -7.6)
  dimension "d14" = 7.62
  dimension "d15" = 7.62
  dimension "d16" = 7.62
  constraint horizontal L671
  constraint vertical L672
  constraint horizontal L673
  constraint vertical L674
  constraint horizontal L675
  constraint perpendicular L675 L676
  constraint parallel L675 L677
  constraint parallel L676 L678
  constraint coincident L679 P4
  constraint coincident L680 P4
  constraint coincident P4 L516.start
  constraint horizontal L681
  constraint perpendicular L681 L682
  constraint parallel L681 L683
  constraint parallel L682 L684
  constraint coincident L685 P5
  constraint coincident L686 P5
  constraint coincident P5 L528.start
  constraint horizontal L687
  constraint perpendicular L687 L688
  constraint parallel L687 L689
  constraint parallel L688 L690
  constraint coincident L691 P6
  constraint coincident L692 P6
  constraint coincident P6 L522.start
  measures "d14" distance of L676.end L677.end
  measures "d15" distance of L682.end L683.end
  measures "d16" distance of L688.end L689.end
extrude "Extrude1" add sketch "Sketch1" along normal blind 1.6 contours L39 L40 L43 | L41 L42 L43 | L63 L64 L65 L66 L67 L68 L69 L70 | L71 L72 L73 | L77 L82 L83 L84 L85 L86 L87 L88 L89 L90 | L126 L127 L128 | L124 L125 L128 | L131 L132 L133 | L129 L130 L133 | L142 L143 L144 L145 L146 L147 L148 L149 L150 L151 | L134 L135 L136 L137 L138 L139 L140 L141 L142 L151 | L169 L170 L171 L172 L173 L174 L175 L176 L177 L178 L179 L180 L181 L182 L183 L184 | L192 L193 L194 L195 L196 L197 L198 L199 L200 L201 | L225 L226 L227 L228 L229 L230 L231 L232 L233 L234 | L217 L218 L219 L220 L221 L222 L223 L224 L225 L234 | L270 L271 L272 L273 L274 L275 L276 L277 L278 L279 | L262 L263 L264 L265 L266 L267 L268 L269 L270 L279 | L293 L294 L295 L296 L297 L298 L299 L300 L301 L302 L303 L304 L305 L306 L307 L308 | L328 L329 L330 L331 L332 L333 L334 L335 L336 L337 | L369 L370 L371 L372 L373 L374 L375 L376 L377 L378 | L361 L362 L363 L364 L365 L366 L367 L368 L369 L378 | L392 L393 L394 L395 L396 L397 L398 L399 L400 L401 L402 L403 L404 L405 L406 L407 | L434 L435 L436 L437 L438 L439 L440 L441 L442 L443 L444 L445 | L446 L447 L448 L449 L450 L451 L452 L453 L454 L455 L456 L457 | L473 L474 L475 L476 L477 L478 L479 L480 L481 L482 | L465 L466 L467 L468 L469 L470 L471 L472 L473 L482 | L496 L497 L498 L499 L500 L501 L502 L503 L504 L505 L506 L507 L508 L509 L510 L511 | L515 L517 L675 L676 L677 L678 | L515 L517 L518 L519 L520 L676 L677 L678 | L521 L523 L687 L688 L689 L690 | L521 L523 L524 L525 L526 L688 L689 L690 | L527 L529 L681 L682 L683 L684 | L527 L529 L530 L531 L532 L682 L683 L684 | L533 L534 A0 L535 L536 A1 A2 L537 A5 | L539 L540 L541 L542 L543 L544 L545 L546 L547 L548 | L585 L586 L587 L588 L589 L590 L591 L592 L593 L594 L595 L596 | L643 L644 L645 L646 L647 L648 L649 L650 L651 L652 L653 L654 | L665 L666 L667 L670 L671 L673 L674 | L667 L668 L669 L671 L672 L673
extrude "Extrude2" add sketch "Sketch1" against normal blind 2.54 contours L665 L666 L667 L670 L671 L673 L674 | L667 L668 L669 L671 L672 L673
sketch "Sketch2" plane through (0, -2.54, 0) normal (0, -1, 0) x (1, 0, 0)
  line L0 (27.705, 3.53) -> (14.885, 3.53)
  line L1 (14.885, 3.53) -> (14.885, 0.87)
  line L2 (14.885, 0.87) -> (27.705, 0.87)
  line L3 (27.705, 0.87) -> (27.705, 3.53)
  line L4 (14.885, 0.87) -> (27.705, 0.87)
  circle A0 centre (26.375, 2.2) radius 1.33
  line L5 (26.025, 2.55) -> (26.725, 2.55)
  line L6 (26.725, 2.55) -> (26.725, 1.85)
  line L7 (26.725, 1.85) -> (26.025, 1.85)
  line L8 (26.025, 1.85) -> (26.025, 2.55)
  line L9 (26.025, 2.55) -> (26.725, 1.85) construction
  line L10 (26.725, 2.55) -> (26.025, 1.85) construction
  line L11 (23.485, 1.85) -> (23.485, 2.55)
  line L12 (24.185, 1.85) -> (23.485, 1.85)
  line L13 (24.185, 2.55) -> (24.185, 1.85)
  line L14 (23.485, 2.55) -> (24.185, 2.55)
  line L15 (20.945, 1.85) -> (20.945, 2.55)
  line L16 (21.645, 1.85) -> (20.945, 1.85)
  line L17 (21.645, 2.55) -> (21.645, 1.85)
  line L18 (20.945, 2.55) -> (21.645, 2.55)
  line L19 (18.405, 1.85) -> (18.405, 2.55)
  line L20 (19.105, 1.85) -> (18.405, 1.85)
  line L21 (19.105, 2.55) -> (19.105, 1.85)
  line L22 (18.405, 2.55) -> (19.105, 2.55)
  line L23 (15.865, 1.85) -> (15.865, 2.55)
  line L24 (16.565, 1.85) -> (15.865, 1.85)
  line L25 (16.565, 2.55) -> (16.565, 1.85)
  line L26 (15.865, 2.55) -> (16.565, 2.55)
  point P0 (26.375, 2.2)
  dimension "d5" = 0.7
  dimension "d6" = 0.7
  dimension "d9" = -10.16
  dimension "d10" = 0
  constraint tangent L4 A0
  constraint tangent L3 A0
  constraint tangent L0 A0
  constraint horizontal L5
  constraint perpendicular L5 L6
  constraint parallel L5 L7
  constraint parallel L6 L8
  constraint coincident L9 P0
  constraint coincident L10 P0
  constraint coincident P0 A0.centre
  measures "d5" distance of L6.end L7.end
  measures "d6" distance of L5.end L6.end
extrude "Extrude3" add sketch "Sketch2" along normal blind 6 contours L5 L6 L7 L8 | L11 L12 L13 L14 | L15 L16 L17 L18 | L19 L20 L21 L22 | L23 L24 L25 L26
chamfer "Chamfer1" distance 0.2 angle 45 20 edges at (26.025, -8.54, 2.2) (26.375, -8.54, 2.55) (26.725, -8.54, 2.2) (26.375, -8.54, 1.85) (23.835, -8.54, 1.85) (24.185, -8.54, 2.2) (23.835, -8.54, 2.55) (23.485, -8.54, 2.2) (21.645, -8.54, 2.2) (21.295, -8.54, 1.85) (21.295, -8.54, 2.55) (20.945, -8.54, 2.2) (19.105, -8.54, 2.2) (18.755, -8.54, 1.85) (18.755, -8.54, 2.55) (18.405, -8.54, 2.2) (16.565, -8.54, 2.2) (16.215, -8.54, 1.85) (15.865, -8.54, 2.2) (16.215, -8.54, 2.55)
extrude "Extrude4" add sketch "Sketch1" along normal up to surface (4.14 mm away) contours L515 L517 L675 L676 L677 L678 | L521 L523 L687 L688 L689 L690 | L527 L529 L681 L682 L683 L684
sketch "Sketch3" plane through (0, 4.14, 0) normal (0, 1, 0) x (-1, 0, 0)
  line L0 (-4.19, 8.83) -> (-11.81, 8.83)
  line L1 (-11.81, 8.83) -> (-11.81, 6.37)
  line L2 (-11.81, 6.37) -> (-4.19, 6.37)
  line L3 (-4.19, 6.37) -> (-4.19, 8.83)
  line L4 (-40.2, 6.37) -> (-29, 6.37)
  line L5 (-40.2, 20.57) -> (-40.2, 6.37)
  line L6 (-29, 20.57) -> (-40.2, 20.57)
  line L7 (-29, 6.37) -> (-29, 20.57)
  line L8 (-26.9, 20.57) -> (-26.9, 6.37)
  line L9 (-15.7, 20.57) -> (-26.9, 20.57)
  line L10 (-15.7, 6.37) -> (-15.7, 20.57)
  line L11 (-26.9, 6.37) -> (-15.7, 6.37)
  line L12 (-2.4, 20.57) -> (-13.6, 20.57)
  line L13 (-13.6, 20.57) -> (-13.6, 6.37)
  line L14 (-2.4, 6.37) -> (-2.4, 20.57)
  line L15 (-13.6, 6.37) -> (-2.4, 6.37)
extrude "Extrude5" add sketch "Sketch3" along normal blind 2.16
equation "d9 = ( -2.54 * 4 ) * 1 mm"
equation "d14 = ( 2.54 * 3 ) * 1 mm"
equation "d15 = ( 2.54 * 3 ) * 1 mm"
equation "d16 = ( 2.54 * 3 ) * 1 mm"
equation "d19 = 4.70 mm - 2.54 mm"
named bodies: "Button PCB"
